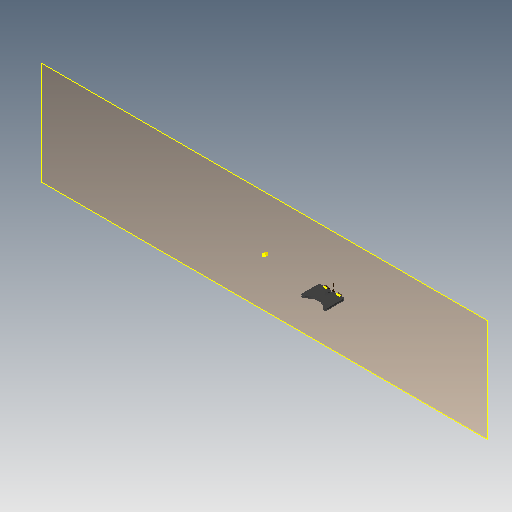
# Autodesk Inventor part: Fanmount_CPY1_CPY_CPY_CPY
Saved by Autodesk Inventor 2017 (Build 210142000, 142)
## iProperties
Created: 2016-07-01
Part Number: Fanmount_CPY1_CPY_CPY_CPY
Material: Acetal Resin, Black
Document SubType Name: Modeling
Designer: User
Density: 1.425 g/cm^3
Appearance: Smooth - Black
Mass: 4.16957 g
Surface Area: 25.5808 cm^2
Volume: 2.92601 cm^3
Author: joshmamo
Autodesk Inventor part; units mm, degrees
ref_plane "YZ Plane" through (0, 0, 0) normal (1, 0, 0) x (0, 1, 0)
ref_plane "XZ Plane" through (0, 0, 0) normal (0, 1, 0) x (-1, 0, 0)
ref_plane "XY Plane" through (0, 0, 0) normal (0, 0, 1) x (1, 0, 0)
ref_plane "Work Plane1" through (0, 0, 0) normal (0, 0, 1) x (1, 0, 0)
sketch "Sketch1" plane through (0, 0, 0) normal (0, 0, 1) x (1, 0, 0)
  line L0 (96.063, 0.903) -> (102.063, 0.903)
  line L1 (102.063, 0.903) -> (102.063, 3.903)
  line L2 (102.063, 3.903) -> (96.063, 3.903)
  line L3 (96.063, 3.903) -> (96.063, 0.903)
  line L4 (96.063, 0.903) -> (102.063, 3.903) construction
  line L5 (102.063, 0.903) -> (96.063, 3.903) construction
  line L6 (117.163, 0.353) -> (117.163, 4.453) projected
  line L7 (123.363, 4.453) -> (123.363, 0.353) projected
  line L8 (117.163, 2.403) -> (123.363, 2.403)
  line L9 (117.263, 3.903) -> (123.263, 3.903)
  line L10 (123.263, 3.903) -> (123.263, 0.903)
  line L11 (123.263, 0.903) -> (117.263, 0.903)
  line L12 (117.263, 0.903) -> (117.263, 3.903)
  line L13 (117.263, 3.903) -> (123.263, 0.903) construction
  line L14 (123.263, 3.903) -> (117.263, 0.903) construction
  point P0 (0, 0)
  point P1 (99.063, 2.403)
  point P2 (120.263, 2.403)
  dimension "d0" = 6
  dimension "d1" = 3
  dimension "d2" = 6
  dimension "d3" = 3
  constraints: 26 end point, 7 midpoint, 4 parallel, 2 horizontal, 2 perpendicular, 1 other
  measures "d0" distance of L2.end L1.end
  measures "d1" distance of L1.end L0.end
  measures "d2" distance of L10.end L11.end
  measures "d3" distance of L9.end L10.end
extrude "Extrusion1" add sketch "Sketch1" against normal blind 3
sketch "Sketch2" plane through (0, 0, 0) normal (0, 0, 1) x (1, 0, 0)
  line L0 (96.063, 0.903) -> (102.063, 0.903) projected
  line L1 (102.063, 0.903) -> (102.063, 3.903) projected
  line L2 (102.063, 3.903) -> (96.063, 3.903) projected
  line L3 (96.063, 3.903) -> (96.063, 0.903) projected
  line L4 (117.263, 3.903) -> (123.263, 3.903) projected
  line L5 (117.263, 0.903) -> (117.263, 3.903) projected
  line L6 (123.263, 0.903) -> (117.263, 0.903) projected
  line L7 (123.263, 3.903) -> (123.263, 0.903) projected
  point P0 (0, 0)
sketch "Sketch3" plane through (0, 0, 0) normal (0, 0, 1) x (1, 0, 0)
  line L0 (89.663, 3.903) -> (129.663, 3.903)
  line L1 (129.663, 3.903) -> (129.663, 0.903)
  line L2 (129.663, 0.903) -> (89.663, 0.903)
  line L3 (89.663, 0.903) -> (89.663, 3.903)
  line L4 (89.663, 3.903) -> (129.663, 0.903) construction
  line L5 (129.663, 3.903) -> (89.663, 0.903) construction
  point P0 (0, 0)
  point P1 (109.663, 2.403)
  dimension "d6" = 40
  dimension "d7" = 3
  constraints: 12 end point, 2 midpoint, 2 parallel, 1 horizontal, 1 perpendicular, 1 other
  measures "d6" distance of L1.end L2.end
  measures "d7" distance of L0.end L1.end
extrude "Extrusion2" add sketch "Sketch3" along normal blind 60
sketch "Sketch4" plane through (96.063, 3.903, -3) normal (0, 1, 0) x (1, 0, 0)
  line L0 (-6.4, -63) -> (33.6, -63) projected
  line L1 (33.6, -3) -> (33.6, -63) projected
  line L2 (-6.4, -63) -> (33.6, -63)
  line L3 (33.6, -63) -> (33.6, -23)
  line L4 (33.6, -23) -> (-6.4, -23)
  line L5 (-6.4, -23) -> (-6.4, -63)
  circle A0 centre (13.6, -43) radius 19
  line L6 (13.6, -43) -> (13.6, -27)
  line L7 (13.6, -27) -> (-2.4, -27)
  circle A1 centre (-2.4, -27) radius 1.6
  circle A2 centre (29.6, -27) radius 1.6
  line L8 (13.6, -43) -> (17.3038, -43)
  circle A3 centre (-2.4, -59) radius 1.6
  circle A4 centre (29.6, -59) radius 1.6
  point P0 (-96.063, -3)
  dimension "d10" = 40
  dimension "d11" = 38
  dimension "d12" = 16
  dimension "d13" = 16
  dimension "d14" = 3.2
  constraints: 14 end point, 5 centre point, 3 perpendicular, 3 symmetric about line, 2 horizontal, 2 parallel, 1 coincident, 1 point on line, 3 other
  measures "d10" distance of L3.end L2.end
  measures "d11" diameter of A0
  measures "d12" distance of L6.start L6.end
  measures "d13" distance of L6.end L7.end
  measures "d14" diameter of A1
extrude "Extrusion3" cut sketch "Sketch4" against normal through all contours A0 | A1 | A2 | A3 | A4
fillet "Fillet1" radius 2 2 edges at (89.663, 2.403, 60) (129.663, 2.403, 60)
sketch "Sketch5" plane through (117.263, 3.903, -3) normal (0, 1, 0) x (1, 0, 0)
  line L0 (-41.845, -71.0861) -> (34.1344, -71.0861)
  line L1 (34.1344, -71.0861) -> (34.1344, -32.9739)
  line L2 (34.1344, -32.9739) -> (-41.845, -32.9739)
  line L3 (-41.845, -32.9739) -> (-41.845, -71.0861)
  point P0 (-117.263, -3)
  constraints: 8 end point, 2 parallel, 1 horizontal, 1 perpendicular
extrude "Extrusion4" cut sketch "Sketch5" against normal blind 40
fillet "Fillet2" radius 2 4 edges at (93.5237, 2.403, 29.9739) (125.8023, 2.403, 29.9739) (129.663, 2.403, 29.9739) (89.663, 2.403, 29.9739)
sketch "Sketch6" plane through (117.263, 3.903, -3) normal (0, 1, 0) x (1, 0, 0)
  line L0 (-9.2, 0) -> (-9.2, -3)
  line L1 (-6, 0) -> (-6, -3)
  line L2 (38.3326, -3) -> (-143.1956, -3) projected
  line L3 (0, -3) -> (-15.2, -3) projected
  line L4 (-7.6, -3) -> (-6.1, -3)
  line L5 (-6.1, -13.7) -> (-7.6, -13.7)
  line L6 (-7.6, -3) -> (-9.1, -3)
  line L7 (-9.1, -13.7) -> (-7.6, -13.7)
  line L8 (-9.1, -3) -> (-9.1, -9)
  line L9 (-9.1, -9) -> (-10.3, -9)
  line L10 (-10.3, -9) -> (-10.3, -11)
  line L11 (-10.3, -11) -> (-9.1, -11)
  line L12 (-9.1, -3) -> (-9.1, -9)
  line L13 (-9.1, -11) -> (-9.1, -13.7)
  line L14 (-7.6, -3) -> (-7.6, -5.4805)
  line L15 (-6.1, -3) -> (-6.1, -9)
  line L16 (-6.1, -9) -> (-4.9, -9)
  line L17 (-4.9, -9) -> (-4.9, -11)
  line L18 (-4.9, -11) -> (-6.1, -11)
  line L19 (-6.1, -11) -> (-6.1, -13.7)
  point P0 (-117.263, -3)
  dimension "d21" = 1.5
  dimension "d22" = 10.7
  dimension "d23" = 1.5
  dimension "d24" = 6
  dimension "d25" = 1.2
  dimension "d26" = 2
  constraints: 36 end point, 2 point on line, 1 midpoint
  measures "d21" distance of L5.start L5.end
  measures "d22" distance of L4.end L5.start
  measures "d23" distance of L5.end L7.start
  measures "d24" distance of L6.end L8.end
  measures "d25" distance of L11.end L10.end
  measures "d26" distance of L10.end L9.end
extrude "Extrusion5" cut sketch "Sketch6" against normal through all
sketch "Sketch7" plane through (0, 0, -3) normal (0, 0, -1) x (-1, 0, 0)
  point P0 (0, 0)
  point P1 (-109.663, 2.403)
body "Solid1"
